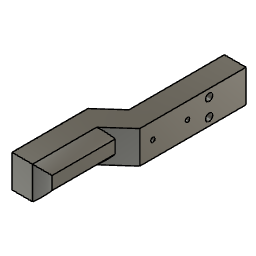
mors_droit (Autodesk Fusion 360 design; units mm, degrees)
Autodesk Fusion 360 part; units mm, degrees
sketch "Esquisse2" plane through (0, 0, 0) normal (0, 0, 1) x (1, 0, 0)
  line L0 (0, 0) -> (10, 0)
  line L1 (10, 0) -> (10, 30)
  line L2 (0, 0) -> (0, 35)
  line L3 (20, 39) -> (20, 88)
  line L4 (20, 88) -> (10, 88)
  line L5 (10, 88) -> (10, 44)
  line L6 (0, 35) -> (10, 44)
  line L7 (10, 30) -> (20, 39)
  dimension "d1" = 10
  dimension "d2" = 30
  dimension "d3" = 35
  dimension "d6" = 10
  dimension "d8" = 10
  dimension "d9" = 14
  dimension "d118" = 49
  constraint coincident L0.start L2.start
  constraint horizontal L0
  constraint perpendicular L0 L1
  constraint perpendicular L0 L2
  constraint perpendicular L3 L4
  constraint perpendicular L4 L5
  constraint parallel L6 L7
  measures "d1" distance of L0.start L0.end
  measures "d2" distance of L0.end L1.end
  measures "d3" distance of L0.start L2.end
  measures "d6" distance of L3.end L4.end
  measures "d8" horizontal distance of L1.end L3.start
  measures "d9" distance of L1.end L5.end
  measures "d118" distance of L3.start L4
extrude "Extrusion1" add sketch "Esquisse2" along normal blind 15
move_face "DécalerLesFaces1" offset 4 1 faces at (10, 10, 10)
fillet "Congé1" radius 4.5 tangency weight 0.1 3 edges at (14, 16.8, 15) (14, 0, 7.5) (14, 16.8, 0)
sketch "Esquisse3" plane through (20, 0, 0) normal (1, 0, 0) x (0, 1, 0)
  line L0 (39, 0) -> (88, 0)
  line L1 (88, 0) -> (88, 15)
  line L2 (88, 15) -> (39, 15)
  line L3 (39, 15) -> (39, 0)
  circle A0 centre (71, 3.5) radius 1.65
  circle A1 centre (71, 11.5) radius 1.65
  circle A2 centre (45, 7.5) radius 1
  circle A3 centre (61, 7.5) radius 1
  line L4 (67, 15) -> (67, 0)
  line L5 (61, 7.5) -> (45, 7.5)
  line L6 (67, 7.5) -> (39, 7.5)
  dimension "d17" = 3.3
  dimension "d19" = 3.3
  dimension "d20" = 17
  dimension "d21" = 17
  dimension "d61" = 2
  dimension "d62" = 2
  dimension "d63" = 16
  dimension "d115" = 7.5
  dimension "d117" = 28
  constraint coincident L2 L4.start
  constraint coincident L0 L4.end
  constraint perpendicular L0 L4
  constraint coincident A3.centre L5.start
  constraint coincident A2.centre L5.end
  constraint coincident L4 L6.start
  constraint coincident L3 L6.end
  constraint perpendicular L3 L6
  constraint midpoint L5 L6
  measures "d17" diameter of A0
  measures "d19" diameter of A1
  measures "d20" distance of L1 A0.centre
  measures "d21" distance of L1 A1.centre
  measures "d61" diameter of A2
  measures "d62" diameter of A3
  measures "d63" distance of A2.centre A3.centre
  measures "d115" distance of L2 A3.centre
  measures "d117" distance of L3 L4
extrude "Extrusion8" cut sketch "Esquisse3" against normal blind 15 contours A0 | A1
extrude "Extrusion11" cut sketch "Esquisse3" against normal blind 8 contours A2 L5 L6 | A2 L5 L6 | A3 L5 L6 | A3 L5 L6
extrude "Extrusion12" add 1 faces at (13.3333, 88, 10) along direction (0, 1, 0) blind 1
sketch "Esquisse8" plane through (0, 0, 0) normal (-1, 0, 0) x (0, -1, 0)
  line L0 (-35, 0) -> (0, 0)
  line L1 (0, 0) -> (0, 15)
  line L2 (0, 15) -> (-35, 15)
  line L3 (-35, 15) -> (-35, 0)
  circle A0 centre (-32.5, 2.5) radius 2.5
  circle A1 centre (-27.5, 2.5) radius 2.5
  circle A2 centre (-22.5, 2.5) radius 2.5
  circle A3 centre (-17.5, 2.5) radius 2.5
  circle A4 centre (-12.5, 2.5) radius 2.5
  circle A5 centre (-7.5, 2.5) radius 2.5
  circle A6 centre (-2.5, 2.5) radius 2.5
  circle A7 centre (-22.5, 2.5) radius 2.5
  circle A8 centre (-32.5, 2.5) radius 2.5
  circle A9 centre (-27.5, 2.5) radius 2.5
  circle A10 centre (-2.5, 2.5) radius 2.5
  line L4 (-35, 15) -> (-35, 0)
  circle A11 centre (-17.5, 2.5) radius 2.5
  line L5 (0, 0) -> (0, 15)
  circle A12 centre (-12.5, 2.5) radius 2.5
  circle A13 centre (-7.5, 2.5) radius 2.5
  line L6 (-35, 0) -> (0, 0)
  circle A14 centre (-17.5, 2.5) radius 2.5
  circle A15 centre (-27.5, 2.5) radius 2.5
  circle A16 centre (-22.5, 2.5) radius 2.5
  circle A17 centre (-2.5, 2.5) radius 2.5
  line L7 (-35, 0) -> (0, 0)
  circle A18 centre (-17.5, 2.5) radius 2.5
  circle A19 centre (-7.5, 2.5) radius 2.5
  circle A20 centre (-12.5, 2.5) radius 2.5
  line L8 (-35, 0) -> (0, 0)
  circle A21 centre (-22.5, 2.5) radius 2.5
  circle A22 centre (-12.5, 2.5) radius 2.5
  circle A23 centre (-32.5, 2.5) radius 2.5
  circle A24 centre (-27.5, 2.5) radius 2.5
  circle A25 centre (-2.5, 2.5) radius 2.5
  circle A26 centre (-32.5, 2.5) radius 2.5
  circle A27 centre (-7.5, 2.5) radius 2.5
  circle A28 centre (-27.5, 7.5) radius 2.5
  circle A29 centre (-22.5, 7.5) radius 2.5
  circle A30 centre (-7.5, 7.5) radius 2.5
  circle A31 centre (-27.5, 7.5) radius 2.5
  circle A32 centre (-32.5, 7.5) radius 2.5
  circle A33 centre (-2.5, 7.5) radius 2.5
  circle A34 centre (-27.5, 7.5) radius 2.5
  circle A35 centre (-17.5, 7.5) radius 2.5
  circle A36 centre (-12.5, 7.5) radius 2.5
  circle A37 centre (-7.5, 7.5) radius 2.5
  circle A38 centre (-22.5, 7.5) radius 2.5
  circle A39 centre (-12.5, 7.5) radius 2.5
  circle A40 centre (-12.5, 7.5) radius 2.5
  circle A41 centre (-17.5, 7.5) radius 2.5
  circle A42 centre (-32.5, 7.5) radius 2.5
  circle A43 centre (-22.5, 7.5) radius 2.5
  circle A44 centre (-2.5, 7.5) radius 2.5
  circle A45 centre (-17.5, 7.5) radius 2.5
  circle A46 centre (-2.5, 7.5) radius 2.5
  circle A47 centre (-12.5, 7.5) radius 2.5
  circle A48 centre (-32.5, 7.5) radius 2.5
  circle A49 centre (-17.5, 7.5) radius 2.5
  circle A50 centre (-2.5, 7.5) radius 2.5
  circle A51 centre (-22.5, 7.5) radius 2.5
  circle A52 centre (-27.5, 7.5) radius 2.5
  circle A53 centre (-7.5, 7.5) radius 2.5
  circle A54 centre (-7.5, 7.5) radius 2.5
  circle A55 centre (-32.5, 7.5) radius 2.5
  circle A56 centre (-27.5, 12.5) radius 2.5
  circle A57 centre (-22.5, 12.5) radius 2.5
  circle A58 centre (-7.5, 12.5) radius 2.5
  circle A59 centre (-27.5, 12.5) radius 2.5
  circle A60 centre (-32.5, 12.5) radius 2.5
  circle A61 centre (-2.5, 12.5) radius 2.5
  circle A62 centre (-27.5, 12.5) radius 2.5
  circle A63 centre (-17.5, 12.5) radius 2.5
  circle A64 centre (-12.5, 12.5) radius 2.5
  circle A65 centre (-7.5, 12.5) radius 2.5
  circle A66 centre (-22.5, 12.5) radius 2.5
  circle A67 centre (-12.5, 12.5) radius 2.5
  circle A68 centre (-12.5, 12.5) radius 2.5
  circle A69 centre (-17.5, 12.5) radius 2.5
  circle A70 centre (-32.5, 12.5) radius 2.5
  circle A71 centre (-22.5, 12.5) radius 2.5
  circle A72 centre (-2.5, 12.5) radius 2.5
  circle A73 centre (-17.5, 12.5) radius 2.5
  circle A74 centre (-2.5, 12.5) radius 2.5
  circle A75 centre (-12.5, 12.5) radius 2.5
  circle A76 centre (-32.5, 12.5) radius 2.5
  circle A77 centre (-17.5, 12.5) radius 2.5
  circle A78 centre (-2.5, 12.5) radius 2.5
  circle A79 centre (-22.5, 12.5) radius 2.5
  circle A80 centre (-27.5, 12.5) radius 2.5
  circle A81 centre (-7.5, 12.5) radius 2.5
  circle A82 centre (-7.5, 12.5) radius 2.5
  circle A83 centre (-32.5, 12.5) radius 2.5
  point P0 (-22.5, 2.5)
  point P1 (-2.5, 2.5)
  point P2 (-32.5, 2.5)
  point P3 (-7.5, 2.5)
  point P4 (-17.5, 2.5)
  point P5 (-12.5, 2.5)
  point P6 (-27.5, 2.5)
  point P7 (-22.5, 2.5)
  point P8 (-17.5, 2.5)
  point P9 (-12.5, 2.5)
  point P10 (-27.5, 2.5)
  point P11 (-7.5, 2.5)
  point P12 (-2.5, 2.5)
  point P13 (-32.5, 2.5)
  point P14 (-27.5, 2.5)
  point P15 (-2.5, 2.5)
  point P16 (-22.5, 2.5)
  point P17 (-12.5, 2.5)
  point P18 (-7.5, 2.5)
  point P19 (-17.5, 2.5)
  point P20 (-32.5, 2.5)
  point P21 (-22.5, 2.5)
  point P22 (-17.5, 2.5)
  point P23 (-12.5, 2.5)
  point P24 (-27.5, 2.5)
  point P25 (-7.5, 2.5)
  point P26 (-2.5, 2.5)
  point P27 (-32.5, 2.5)
  point P28 (-27.5, 7.5)
  point P29 (-2.5, 7.5)
  point P30 (-22.5, 7.5)
  point P31 (-12.5, 7.5)
  point P32 (-7.5, 7.5)
  point P33 (-17.5, 7.5)
  point P34 (-32.5, 7.5)
  point P35 (-7.5, 7.5)
  point P36 (-32.5, 7.5)
  point P37 (-2.5, 7.5)
  point P38 (-22.5, 7.5)
  point P39 (-17.5, 7.5)
  point P40 (-12.5, 7.5)
  point P41 (-27.5, 7.5)
  point P42 (-7.5, 7.5)
  point P43 (-2.5, 7.5)
  point P44 (-32.5, 7.5)
  point P45 (-22.5, 7.5)
  point P46 (-12.5, 7.5)
  point P47 (-27.5, 7.5)
  point P48 (-27.5, 7.5)
  point P49 (-7.5, 7.5)
  point P50 (-22.5, 7.5)
  point P51 (-17.5, 7.5)
  point P52 (-2.5, 7.5)
  point P53 (-12.5, 7.5)
  point P54 (-17.5, 7.5)
  point P55 (-32.5, 7.5)
  point P56 (-27.5, 12.5)
  point P57 (-2.5, 12.5)
  point P58 (-22.5, 12.5)
  point P59 (-12.5, 12.5)
  point P60 (-7.5, 12.5)
  point P61 (-17.5, 12.5)
  point P62 (-32.5, 12.5)
  point P63 (-7.5, 12.5)
  point P64 (-32.5, 12.5)
  point P65 (-2.5, 12.5)
  point P66 (-22.5, 12.5)
  point P67 (-17.5, 12.5)
  point P68 (-12.5, 12.5)
  point P69 (-27.5, 12.5)
  point P70 (-7.5, 12.5)
  point P71 (-2.5, 12.5)
  point P72 (-32.5, 12.5)
  point P73 (-22.5, 12.5)
  point P74 (-12.5, 12.5)
  point P75 (-27.5, 12.5)
  point P76 (-27.5, 12.5)
  point P77 (-7.5, 12.5)
  point P78 (-22.5, 12.5)
  point P79 (-17.5, 12.5)
  point P80 (-2.5, 12.5)
  point P81 (-12.5, 12.5)
  point P82 (-17.5, 12.5)
  point P83 (-32.5, 12.5)
  constraint tangent L1 A6
  constraint tangent A10 L5
extrude "Extrusion13" add sketch "Esquisse8" along normal blind 1 draft -70 contours A60 A70 A76 A83
extrude "Extrusion14" add sketch "Esquisse8" along normal blind 1 draft -70 contours A56 A59 A62 A80
extrude "Extrusion15" add sketch "Esquisse8" along normal blind 1 draft -70 contours A57 A66 A71 A79
extrude "Extrusion16" add sketch "Esquisse8" along normal blind 1 draft -70 contours A63 A69 A73 A77
extrude "Extrusion17" add sketch "Esquisse8" along normal blind 1 draft -70 contours A64 A67 A68 A75
extrude "Extrusion18" add sketch "Esquisse8" along normal blind 1 draft -70 contours A58 A65 A81 A82
extrude "Extrusion19" add sketch "Esquisse8" along normal blind 1 draft -70 contours A61 A72 A74 A78
extrude "Extrusion20" add sketch "Esquisse8" along normal blind 1 draft -70 contours A32 A42 A48 A55
extrude "Extrusion21" add sketch "Esquisse8" along normal blind 1 draft -70 contours A28 A31 A34 A52
extrude "Extrusion22" add sketch "Esquisse8" along normal blind 1 draft -70 contours A29 A38 A43 A51
extrude "Extrusion23" add sketch "Esquisse8" along normal blind 1 draft -70 contours A35 A41 A45 A49
extrude "Extrusion24" add sketch "Esquisse8" along normal blind 1 draft -70 contours A36 A39 A40 A47
extrude "Extrusion25" add sketch "Esquisse8" along normal blind 1 draft -70 contours A30 A37 A53 A54
extrude "Extrusion26" add sketch "Esquisse8" along normal blind 1 draft -70 contours A33 A44 A46 A50
extrude "Extrusion27" add sketch "Esquisse8" along normal blind 1 draft -70 contours A0 A8 A23 A26
extrude "Extrusion28" add sketch "Esquisse8" along normal blind 1 draft -70 contours A1 A9 A15 A24
extrude "Extrusion29" add sketch "Esquisse8" along normal blind 1 draft -70 contours A2 A7 A16 A21
extrude "Extrusion30" add sketch "Esquisse8" along normal blind 1 draft -70 contours A3 A11 A14 A18
extrude "Extrusion31" add sketch "Esquisse8" along normal blind 1 draft -70 contours A4 A12 A20 A22
extrude "Extrusion32" add sketch "Esquisse8" along normal blind 1 draft -70 contours A5 A13 A19 A27
extrude "Extrusion33" add sketch "Esquisse8" along normal blind 1 draft -70 contours A6 A10 A17 A25
extrude "Extrusion34" cut 1 faces at (13.3333, 89, 10) along direction (0, -1, 0) blind 1
extrude "Extrusion10" [suppressed]
extrude "Extrusion9" [suppressed]
extrude "Extrusion4" [suppressed]
extrude "Extrusion5" [suppressed]
extrude "Extrusion6" [suppressed]
fillet "Congé3" [suppressed]
extrude "Extrusion7" [suppressed]
fillet "Congé4" [suppressed]
extrude "Extrusion3" [suppressed]
extrude "Extrusion2" [suppressed]
fillet "Congé2" [suppressed]
equation "d19 = d17"
equation "d20 = d21"
